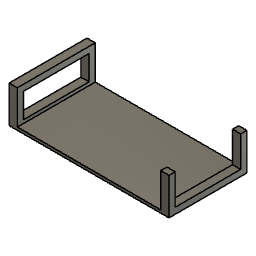
Tissue mount 1.5 arms 20mm v2 (Autodesk Fusion 360 design; units mm, degrees)
Autodesk Fusion 360 part; units mm, degrees
note: some values were not read from the file. Chosen so that the rebuilt part matches the saved one: which bodies a step acts on; which face or edge a step refers to.
sketch "Sketch1" plane through (0, 0, 0) normal (0, 1, 0) x (1, 0, 0)
  line L0 (0, 0) -> (35, 0)
  line L1 (35, 0) -> (35, -9)
  line L2 (35, -9) -> (0, -9)
  line L3 (0, -9) -> (0, 0)
  dimension "d1" = 35
  dimension "d2" = 9
  constraint horizontal L0
  constraint vertical L1
  constraint horizontal L2
  constraint vertical L3
  constraint coincident L0.start L3.end
  measures "d1" distance of L0.start L0.end
  measures "d2" distance of L0.start L2.end
extrude "Extrude1" add sketch "Sketch1" along normal blind 0.5 makes body 1
extrude "Extrude2" add 1 faces at (11.6667, 0.5, 3) along direction (0, 1, 0) blind 0.2 on bodies 1 bodies 1
sketch "Sketch2" plane through (0, 0.7, 0) normal (0, 1, 0) x (-1, 0, 0)
  line L0 (0, 9) -> (-35, 9)
  line L1 (-35, 9) -> (-35, 0)
  line L2 (-35, 0) -> (0, 0)
  line L3 (0, 0) -> (0, 9)
  line L4 (0, 0) -> (-2, 0)
  line L5 (-2, 0) -> (-2, 9)
  line L6 (-2, 9) -> (0, 9)
  line L7 (0, 9) -> (0, 0)
  dimension "d7" = 2
  constraint horizontal L4
  constraint vertical L5
  constraint horizontal L6
  constraint vertical L7
  constraint coincident L2.end L3.start
  measures "d7" distance of L2.end L4.end
extrude "Extrude3" add sketch "Sketch2" along normal blind 8.3 contours L0 L2 L3 L4 L5 L6 L7 bodies 1
sketch "Sketch3" plane through (2, 0, 0) normal (1, 0, 0) x (0, 0, -1)
  line L0 (-9, 0.7) -> (0, 0.7)
  line L1 (0, 0.7) -> (0, 9)
  line L2 (0, 9) -> (-9, 9)
  line L3 (-9, 9) -> (-9, 0.7)
  line L4 (-9, 9) -> (-4.5, 9)
  line L5 (-4.5, 9) -> (-4.5, 4.85)
  line L6 (-4.5, 4.85) -> (-9, 4.85)
  line L7 (-9, 4.85) -> (-9, 9)
  line L8 (-4.5, 9) -> (0, 9)
  line L9 (0, 9) -> (0, 4.85)
  line L10 (0, 4.85) -> (-4.5, 4.85)
  line L11 (-4.5, 4.85) -> (-4.5, 9)
  line L12 (-9, 4.85) -> (-4.5, 4.85)
  line L13 (-4.5, 4.85) -> (-4.5, 0.7)
  line L14 (-4.5, 0.7) -> (-9, 0.7)
  line L15 (-9, 0.7) -> (-9, 4.85)
  line L16 (-4.5, 4.85) -> (0, 4.85)
  line L17 (0, 4.85) -> (0, 0.7)
  line L18 (0, 0.7) -> (-4.5, 0.7)
  line L19 (-4.5, 0.7) -> (-4.5, 4.85)
  circle A0 centre (-6.75, 6.925) radius 0.75
  circle A1 centre (-2.25, 6.925) radius 0.75
  circle A2 centre (-6.75, 2.775) radius 0.75
  circle A3 centre (-2.25, 2.775) radius 0.75
  dimension "d10" = 4.5
  dimension "d11" = 4.15
  dimension "d12" = 1.5
  dimension "d13" = 1.5
  dimension "d14" = 1.5
  dimension "d15" = 1.5
  constraint horizontal L4
  constraint vertical L5
  constraint horizontal L6
  constraint vertical L7
  constraint coincident L2.end L3.start
  constraint horizontal L8
  constraint vertical L9
  constraint horizontal L10
  constraint vertical L11
  constraint midpoint L1 L9.end
  constraint horizontal L12
  constraint vertical L13
  constraint horizontal L14
  constraint vertical L15
  constraint midpoint L0 L13.end
  constraint horizontal L16
  constraint vertical L17
  constraint horizontal L18
  constraint vertical L19
  constraint coincident L0.end L1.start
  measures "d10" distance of L2.end L4.end
  measures "d11" distance of L2.end L6.end
  measures "d12" diameter of A0
  measures "d13" diameter of A1
  measures "d14" diameter of A2
  measures "d15" diameter of A3
extrude "Extrude4" cut sketch "Sketch3" against normal up to surface (2 mm away) contours A0 | A1 | A2 | A3 bodies 1
sketch "Sketch4" plane through (0, 0.7, 0) normal (0, 1, 0) x (-1, 0, 0)
  line L0 (-2, 0) -> (-2, 9)
  line L1 (-2, 9) -> (-35, 9)
  line L2 (-35, 9) -> (-35, 0)
  line L3 (-35, 0) -> (-2, 0)
  line L4 (-35, 9) -> (-33, 9)
  line L5 (-33, 9) -> (-33, 0)
  line L6 (-33, 0) -> (-35, 0)
  line L7 (-35, 0) -> (-35, 9)
  dimension "d18" = 2
  constraint horizontal L4
  constraint vertical L5
  constraint horizontal L6
  constraint vertical L7
  constraint coincident L1.end L2.start
  measures "d18" distance of L1.end L4.end
extrude "Extrude5" add sketch "Sketch4" along normal up to surface (8.3 mm away) contours L1 L2 L3 L4 L5 L6 L7 bodies 1
sketch "Sketch5" plane through (33, 0, 0) normal (-1, 0, 0) x (0, 0, 1)
  line L0 (9, 9) -> (0, 9)
  line L1 (0, 9) -> (0, 0.7)
  line L2 (0, 0.7) -> (9, 0.7)
  line L3 (9, 0.7) -> (9, 9)
  line L4 (6, 3.35) -> (3, 3.35)
  line L5 (3, 3.35) -> (3, 6.35)
  line L6 (3, 6.35) -> (6, 6.35)
  line L7 (6, 6.35) -> (6, 3.35)
  line L8 (6, 3.35) -> (3, 6.35) construction
  line L9 (3, 3.35) -> (6, 6.35) construction
  point P0 (4.5, 4.85)
  point P1 (4.5, 4.85)
  dimension "d21" = 3
  dimension "d22" = 3
  constraint horizontal L4
  constraint perpendicular L4 L5
  constraint parallel L4 L6
  constraint parallel L5 L7
  constraint coincident L8 P1
  constraint coincident L9 P1
  constraint coincident P1 P0
  measures "d21" distance of L5.end L6.end
  measures "d22" distance of L4.end L5.end
extrude "Extrude6" cut sketch "Sketch5" against normal up to surface (2 mm away) contours L4 L5 L6 L7 bodies 1
delete_face "DeleteFace1" 1 faces at (0.6667, 6.8503, 1.5037) on bodies 1
delete_face "DeleteFace2" 1 faces at (0.6667, 6.8503, 6.0037) on bodies 1
delete_face "DeleteFace3" 1 faces at (0.6667, 2.7003, 6.0037) on bodies 1
delete_face "DeleteFace4" 1 faces at (0.6667, 2.7003, 1.5037) on bodies 1
delete_face "DeleteFace5" 1 faces at (33.6667, 4.35, 3) on bodies 1
sketch "Sketch6" plane through (35, 0, 0) normal (1, 0, 0) x (0, 0, -1)
  line L0 (0, 0) -> (0, 9)
  line L1 (0, 9) -> (-9, 9)
  line L2 (-9, 9) -> (-9, 0)
  line L3 (-9, 0) -> (0, 0)
  line L4 (-9, 9) -> (-7.5, 9)
  line L5 (-7.5, 9) -> (-7.5, 7.5)
  line L6 (-7.5, 7.5) -> (-9, 7.5)
  line L7 (-9, 7.5) -> (-9, 9)
  line L8 (0, 9) -> (-1.5, 9)
  line L9 (-1.5, 9) -> (-1.5, 7.5)
  line L10 (-1.5, 7.5) -> (0, 7.5)
  line L11 (0, 7.5) -> (0, 9)
  line L12 (-9, 0) -> (-7.5, 0)
  line L13 (-7.5, 0) -> (-7.5, 1.5)
  line L14 (-7.5, 1.5) -> (-9, 1.5)
  line L15 (-9, 1.5) -> (-9, 0)
  line L16 (0, 0) -> (-1.5, 0)
  line L17 (-1.5, 0) -> (-1.5, 1.5)
  line L18 (-1.5, 1.5) -> (0, 1.5)
  line L19 (0, 1.5) -> (0, 0)
  line L20 (-7.5, 7.5) -> (-1.5, 7.5)
  line L21 (-1.5, 7.5) -> (-1.5, 1.5)
  line L22 (-1.5, 1.5) -> (-7.5, 1.5)
  line L23 (-7.5, 1.5) -> (-7.5, 7.5)
  dimension "d25" = 1.5
  dimension "d26" = 1.5
  dimension "d27" = 1.5
  dimension "d28" = 1.5
  dimension "d29" = 1.5
  dimension "d30" = 1.5
  dimension "d31" = 1.5
  dimension "d32" = 1.5
  constraint horizontal L4
  constraint vertical L5
  constraint horizontal L6
  constraint vertical L7
  constraint coincident L1.end L2.start
  constraint horizontal L8
  constraint vertical L9
  constraint horizontal L10
  constraint vertical L11
  constraint coincident L0.end L1.start
  constraint horizontal L12
  constraint vertical L13
  constraint horizontal L14
  constraint vertical L15
  constraint coincident L2.end L3.start
  constraint horizontal L16
  constraint vertical L17
  constraint horizontal L18
  constraint vertical L19
  constraint coincident L0.start L3.end
  constraint horizontal L20
  constraint vertical L21
  constraint horizontal L22
  constraint vertical L23
  measures "d25" distance of L1.end L4.end
  measures "d26" distance of L1.end L6.end
  measures "d27" distance of L0.end L8.end
  measures "d28" distance of L0.end L10.end
  measures "d29" distance of L2.end L12.end
  measures "d30" distance of L2.end L14.end
  measures "d31" distance of L0.start L16.end
  measures "d32" distance of L0.start L18.end
extrude "Extrude7" cut sketch "Sketch6" against normal up to surface (2 mm away) contours L20 L21 L22 L23 bodies 1
sketch "Sketch7" plane through (0, 0, 0) normal (-1, 0, 0) x (0, 0, 1)
  line L0 (0, 0) -> (9, 0)
  line L1 (9, 0) -> (9, 9)
  line L2 (9, 9) -> (0, 9)
  line L3 (0, 9) -> (0, 0)
  line L4 (0, 9) -> (1.5, 9)
  line L5 (1.5, 9) -> (1.5, 7.5)
  line L6 (1.5, 7.5) -> (0, 7.5)
  line L7 (0, 7.5) -> (0, 9)
  line L8 (9, 9) -> (7.5, 9)
  line L9 (7.5, 9) -> (7.5, 7.5)
  line L10 (7.5, 7.5) -> (9, 7.5)
  line L11 (9, 7.5) -> (9, 9)
  line L12 (0, 0) -> (1.5, 0)
  line L13 (1.5, 0) -> (1.5, 1.5)
  line L14 (1.5, 1.5) -> (0, 1.5)
  line L15 (0, 1.5) -> (0, 0)
  line L16 (9, 0) -> (7.5, 0)
  line L17 (7.5, 0) -> (7.5, 1.5)
  line L18 (7.5, 1.5) -> (9, 1.5)
  line L19 (9, 1.5) -> (9, 0)
  line L20 (1.5, 7.5) -> (7.5, 7.5)
  line L21 (7.5, 7.5) -> (7.5, 1.5)
  line L22 (7.5, 1.5) -> (1.5, 1.5)
  line L23 (1.5, 1.5) -> (1.5, 7.5)
  dimension "d35" = 1.5
  dimension "d36" = 1.5
  dimension "d37" = 1.5
  dimension "d38" = 1.5
  dimension "d39" = 1.5
  dimension "d40" = 1.5
  dimension "d41" = 1.5
  dimension "d42" = 1.5
  constraint horizontal L4
  constraint vertical L5
  constraint horizontal L6
  constraint vertical L7
  constraint coincident L2.end L3.start
  constraint horizontal L8
  constraint vertical L9
  constraint horizontal L10
  constraint vertical L11
  constraint coincident L1.end L2.start
  constraint horizontal L12
  constraint vertical L13
  constraint horizontal L14
  constraint vertical L15
  constraint coincident L0.start L3.end
  constraint horizontal L16
  constraint vertical L17
  constraint horizontal L18
  constraint vertical L19
  constraint coincident L0.end L1.start
  constraint horizontal L20
  constraint vertical L21
  constraint horizontal L22
  constraint vertical L23
  measures "d35" distance of L2.end L4.end
  measures "d36" distance of L2.end L6.end
  measures "d37" distance of L1.end L8.end
  measures "d38" distance of L1.end L10.end
  measures "d39" distance of L0.start L12.end
  measures "d40" distance of L0.start L14.end
  measures "d41" distance of L0.end L16.end
  measures "d42" distance of L0.end L18.end
extrude "Extrude8" cut sketch "Sketch7" against normal up to surface (2 mm away) contours L20 L21 L22 L23 bodies 1
ref_plane "WorkPlane1" through (17.5, 4.5, 4.5) normal (0, 0, 1) x (1, 0, 0)
split "Split1" by plane through (17.5, 4.5, 4.5) normal (0, 0, 1) bodies 1 makes body 2 at (11.6667, 0, 6)
move_body "Move1" bodies 1 to x (1, 0, 0) y (0, 1, 0) z (0, 0, 1) at (0, 0, -10)
extrude "Extrude9" add 3 faces at (0.6667, 0.7333, 4.5) (34.3333, 8, 4.5) (0.6667, 8.5, 4.5) along direction (0, 0, -1) up to surface end surface through (17.5, 4.5, -5.5) normal (0, 0, 1) offset 0 on bodies 2 bodies 2 1
ref_plane "WorkPlane2" through (34, 4.5, -8.5) normal (0, 0, 1) x (0, 1, 0)
ref_plane "WorkPlane3" through (34, 4.5, 7.5) normal (0, 0, -1) x (0, -1, 0)
split "Split2" by plane through (34, 4.5, -8.5) normal (0, 0, 1) and through (34, 4.5, 7.5) normal (0, 0, -1) bodies 2 makes body 3 at (34.3333, 3.2333, -10) makes body 4 at (34.3333, 9, -3.1667) makes body 5 at (23.3333, 0, 2.1667) makes body 6 at (1.3333, 7.5, 2.1667)
delete_body "RemoveBody1" bodies 4
ref_plane "WorkPlane4" through (17.5, 0.75, -0.5) normal (1, 0, 0) x (0, 0, -1)
split "Split3" by plane through (17.5, 0.75, -0.5) normal (1, 0, 0) bodies 3 2 6 5 makes body 9 at (29.1667, 0, 2.1667) makes body 8 at (34.3333, 3.2333, 9) makes body 7 at (34.3333, 3.2333, -10)
ref_plane "WorkPlane5" through (8.75, 4.5, -0.5) normal (0, 0, 1) x (1, 0, 0)
move_body "Move2" bodies 2 3 6 5 to x (1, 0, 0) y (0, 1, 0) z (0, 0, 1) at (-4, 0, 0)
extrude "Extrude10" add 3 faces at (13.5, 0.2333, 8) (13.5, 0.2333, -3.1667) (13.5, 0.4667, -9) along direction (1, 0, 0) up to surface end surface through (17.5, 0.75, -0.5) normal (-1, 0, 0) offset 0 on bodies 2 3 5 bodies 2 6 3 5 7 8 9
combine "Combine1" operation add target body 2 tool bodies 6
